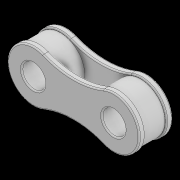
# Autodesk Inventor part: Eslabón Inicial Cadena
Saved by Autodesk Inventor 2021 (Build 250183000, 183)
## iProperties
Created: 2021-04-22
Part Number: Eslabón Inicial Cadena
Material: Generic
Document SubType Name: Modeling
Designer: maaro
Density: 1 g/cm^3
Appearance: Default
p: 12,700 mm
d1: 7,750 mm
d2: 3,660 mm
b1: 3,300 mm
Pt: 13,920 mm
G: 8,200 mm
t: 1,000 mm
d0: 1,650 mm
d3: 8,200 mm
d4: 12,700 mm
d5: 12,500 mm
d6: 3,660 mm
d7: 1,000 mm
d8: 0,00 deg
d9: 7,750 mm
d10: 3,300 mm
d11: 0,00 deg
d12: 0,200 mm
Author: maaro
Autodesk Inventor part; units mm, degrees
ref_plane "YZ Plane" through (0, 0, 0) normal (1, 0, 0) x (0, 1, 0)
ref_plane "XZ Plane" through (0, 0, 0) normal (0, 1, 0) x (-1, 0, 0)
ref_plane "Work Plane1" through (0, 0, 1.65) normal (0, 0, 1) x (1, 0, 0)
sketch "Sketch1" plane through (0, 0, 1.65) normal (0, 0, 1) x (1, 0, 0)
  arc A0 (-4.7816, 3.7882) -> (-4.7816, -3.7882) centre (-6.35, 0) ccw
  arc A1 (4.7816, -3.7882) -> (4.7816, 3.7882) centre (6.35, 0) ccw
  arc A2 (-4.7816, 3.7882) -> (4.7816, 3.7882) centre (0, 15.3375) ccw
  arc A3 (4.7816, -3.7882) -> (-4.7816, -3.7882) centre (0, -15.3375) ccw
  line L0 (-6.35, 0) -> (6.35, 0) construction
  circle A4 centre (-6.35, 0) radius 1.83
  circle A5 centre (6.35, 0) radius 1.83
  point P0 (0, 0)
  point P1 (0, 0)
  dimension "d3" = 8.2
  dimension "d4" = 12.7
  dimension "d5" = 12.5
  dimension "d6" = 3.66
  constraints: 8 point on circle, 6 centre point, 4 tangent, 3 coincident, 3 equal radius, 2 end point, 2 horizontal alignment, 1 horizontal, 1 midpoint
  measures "d3" diameter of A0
  measures "d4" distance of L0.start L0.end
  measures "d5" radius of A2
  measures "d6" diameter of A4
extrude "Extrusion1" add sketch "Sketch1" along normal blind 1
mirror "Mirror1" about plane through (0, 0, 0) normal (0, 0, 1)
sketch "Sketch2" plane through (0, 0, 0) normal (0, 0, 1) x (1, 0, 0)
  circle A0 centre (-6.35, 0) radius 1.83 projected
  circle A1 centre (-6.35, 0) radius 3.875
  circle A2 centre (6.35, 0) radius 1.83 projected
  circle A3 centre (6.35, 0) radius 3.875
  point P0 (0, 0)
  dimension "d9" = 7.75
  constraints: 2 centre point, 2 coincident, 1 equal radius
  measures "d9" diameter of A1
extrude "Extrusion2" add sketch "Sketch2" along normal mid plane 3.3
fillet "Fillet1" radius 0.2 20 edges at (-10.45, 0, 2.65) (0, -2.8375, 2.65) (10.45, 0, 2.65) (0, 2.8375, 2.65) (-10.45, 0, 1.65) (0, -2.8375, 1.65) (10.45, 0, 1.65) (0, 2.8375, 1.65) (-8.18, 0, 2.65) (-10.45, 0, -2.65) (0, -2.8375, -2.65) (10.45, 0, -2.65) (0, 2.8375, -2.65) (-10.45, 0, -1.65) (0, -2.8375, -1.65) (10.45, 0, -1.65) (0, 2.8375, -1.65) (4.52, 0, -2.65) (-8.18, 0, -2.65) (4.52, 0, 2.65)
equation "\"d3\" = G"
equation "\"d4\" = p"
equation "\"d6\" = d2"
equation "\"d7\" = t"
equation "\"d9\" = d1"
equation "\"d10\" = b1"
equation "\"p\" = 12.7"
equation "\"d1\" = 7.75"
equation "\"d2\" = 3.66"
equation "\"b1\" = 3.3"
equation "\"Pt\" = 13.92"
equation "\"d0\" = 0.5 * b1"
equation "\"G\" = 8.2"
equation "\"t\" = 1"
body "Solid1"
